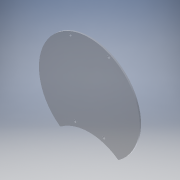
# Autodesk Inventor part: Middle plate
Saved by Autodesk Inventor 2016 (Build 200138000, 138)
## iProperties
Created: 2015-08-24
Part Number: Middle plate
Material: Polycarbonate, Clear
Document SubType Name: Modeling
Designer: TFHulbert
Density: 1.2 g/cm^3
Appearance: Polycarbonate - Clear
Author: TFHulbert
Autodesk Inventor part; units mm, degrees
ref_plane "YZ Plane" through (0, 0, 0) normal (1, 0, 0) x (0, 1, 0)
ref_plane "XZ Plane" through (0, 0, 0) normal (0, 1, 0) x (-1, 0, 0)
ref_plane "XY Plane" through (0, 0, 0) normal (0, 0, 1) x (1, 0, 0)
sketch "Sketch1" plane through (0, 0, 0) normal (0, 1, 0) x (-1, 0, 0)
  arc A0 (56.1004, -98.4936) -> (58.4448, -98.4888) centre (57.2693, -96.8707) ccw
  arc A1 (56.1004, -98.4936) -> (-62.636, -98.4936) centre (-3.2678, -180.9204) ccw
  arc A2 (-64.9803, -98.4888) -> (-62.636, -98.4936) centre (-63.8049, -96.8707) ccw
  circle A3 centre (-33.2678, -74.3391) radius 2.5
  circle A4 centre (26.7322, -74.3391) radius 2.5
  circle A5 centre (-43.2678, 76.4616) radius 2.5
  circle A6 centre (36.7322, 76.4616) radius 2.5
  arc A7 (58.4448, -98.4888) -> (-64.9803, -98.4888) centre (-3.2678, -13.5384) ccw
  circle A8 centre (-33.2678, -74.3391) radius 2.5
  circle A9 centre (26.7322, -74.3391) radius 2.5
  circle A10 centre (-33.2678, -74.3391) radius 2.5
  circle A11 centre (26.7322, -74.3391) radius 2.5
  point P0 (0, 0)
  dimension "d25" = 90
  dimension "d26" = 40
  dimension "d27" = 90
  dimension "d28" = 40
  constraints: 12 centre point, 8 point on circle
  measures "d25" vertical distance of A7.centre A6.centre
  measures "d26" horizontal distance of A7.centre A6.centre
  measures "d27" vertical distance of A7.centre A5.centre
  measures "d28" horizontal distance of A7.centre A5.centre
extrude "Extrusion5" add sketch "Sketch1" along normal blind 3
body "Solid3"
